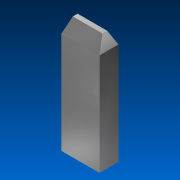
# Autodesk Inventor part: Soanar Power Module Pin B
Saved by Autodesk Inventor 2016 (Build 200138000, 138)
## iProperties
Created: 2013-08-06
Project: Power Entry Module - Soanar PP4003
Material: Nickel-Copper Alloy 400
Description: Soanar Power Module Pin B
Document SubType Name: Modeling
Designer: sdarley
Density: 8.83 g/cm^3
Appearance: Chrome - Polished
Title: Soanar Power Module Pin B
Author: sdarley
Revision Number: 1
Autodesk Inventor part; units mm, degrees
ref_plane "YZ Plane" through (0, 0, 0) normal (1, 0, 0) x (0, 1, 0)
ref_plane "XZ Plane" through (0, 0, 0) normal (0, 1, 0) x (-1, 0, 0)
ref_plane "XY Plane" through (0, 0, 0) normal (0, 0, 1) x (1, 0, 0)
sketch "Sketch1" plane through (0, 0, 0) normal (0, 1, 0) x (-1, 0, 0)
  line L0 (-2, 0) -> (2, 0)
  line L1 (2, 0) -> (2, 12.1)
  line L2 (2, 12.1) -> (-2, 12.1)
  line L3 (-2, 12.1) -> (-2, 0)
  point P0 (0, 0)
  point P1 (0, 0)
  dimension "d0" = 4
  dimension "d1" = 12.1
  constraints: 8 end point, 2 parallel, 1 coincident, 1 horizontal, 1 midpoint, 1 perpendicular
  measures "d0" distance between parallel lines of L1 L3
  measures "d1" distance between parallel lines of L0 L2
extrude "Extrusion1" add sketch "Sketch1" along normal mid plane 2
chamfer "Chamfer1" distance 1.4 distance2 0.45 1 edges at (-2, 0, 12.1) measured on face at (-2, 0.3333, 8.0667)
chamfer "Chamfer2" distance 1.4 distance2 0.45 1 edges at (2, 0, 12.1) measured on face at (2, -0.3333, 8.0667)
chamfer "Chamfer3" distance 1.4 distance2 0.75 1 edges at (0, 1, 12.1) measured on face at (0.6667, 1, 7.1333)
chamfer "Chamfer4" distance 1.4 distance2 0.75 1 edges at (0, -1, 12.1) measured on face at (0.6667, -1, 7.1333)
body "Solid1"
